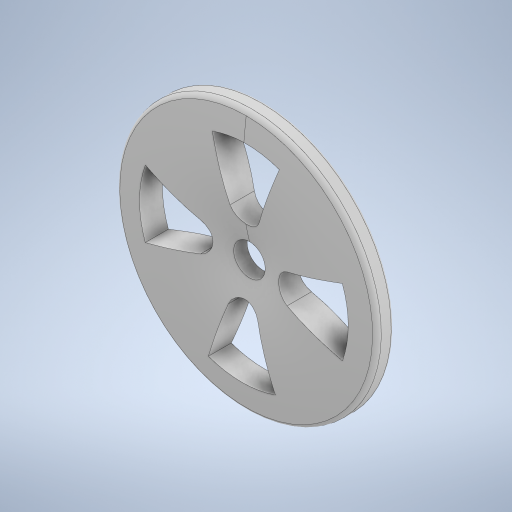
# Autodesk Inventor part: Anti tip wheels
Saved by Autodesk Inventor 2023 (Build 270158000, 158)
## iProperties
Created: 2023-11-13
Part Number: Anti tip wheels
Material: Generic
Document SubType Name: Modeling
Designer: Raghav
Density: 1 g/cm^3
Appearance: Default
Author: Raghav
Autodesk Inventor part; units mm, degrees
ref_plane "YZ Plane" through (0, 0, 0) normal (1, 0, 0) x (0, 1, 0)
ref_plane "XZ Plane" through (0, 0, 0) normal (0, 1, 0) x (-1, 0, 0)
ref_plane "XY Plane" through (0, 0, 0) normal (0, 0, 1) x (1, 0, 0)
sketch "Sketch1" plane through (0, 0, 0) normal (1, 0, 0) x (0, 1, 0)
  line L0 (52.3875, 0) -> (52.3875, 2)
  line L1 (52.3875, 0) -> (52.3875, -2)
  arc A0 (52.3875, 2) -> (50.9047, 4.0295) centre (50.2572, 2) ccw
  arc A1 (51.1141, -2.9824) -> (52.3875, -2) centre (51.3718, -2) ccw
  line L2 (50.9047, 4.0295) -> (25.8188, 7.012) construction
  line L3 (25.8188, 7.012) -> (16.2938, 5.4245) construction
  line L4 (16.2938, 5.4245) -> (-0.0182, 1.08) construction
  spline S0 degree 3 poles (50.9047, 4.0295) (25.8188, 7.012) (16.2938, 5.4245) (-0.0182, 1.08) knots 1 1 1 1 2 2 2 2
  line L5 (0, 0) -> (52.3875, 0)
  line L6 (51.1141, -2.9824) -> (25.8188, -7.012) construction
  line L7 (25.8188, -7.012) -> (16.2938, -5.4245) construction
  line L8 (16.2938, -5.4245) -> (-0.0182, -1.08) construction
  spline S1 degree 3 poles (51.1141, -2.9824) (25.8188, -7.012) (16.2938, -5.4245) (-0.0182, -1.08) knots 1 1 1 1 2 2 2 2
  line L9 (-0.0182, -1.08) -> (-0.0182, 1.08)
  dimension "d0" = 2
  dimension "d1" = 2
  constraints: 8 end point, 4 point on circle, 3 symmetric about line, 3 vertical, 2 centre point, 2 tangent, 1 horizontal, 6 other
  measures "d0" distance of L0.start L0.end
  measures "d1" distance of L0.start L1.end
revolve "Revolution1" add sketch "Sketch1" angle 360 about axis through (0, -0.0182, -1.08) along (0, 0, 1)
sketch "Sketch2" plane through (0, 0, 0) normal (0, 0, 1) x (1, 0, 0)
  circle A0 centre (0, 0) radius 6.35
  constraints: 1 centre point, 1 coincident
extrude "Extrusion1" cut sketch "Sketch2" along normal mid plane 105.25
sketch "Sketch3" plane through (0, 0, 0) normal (0, 0, 1) x (1, 0, 0)
  line L0 (0, 0) -> (-14.2875, -39.6875)
  arc A0 (-14.2875, -39.6875) -> (12.7, -39.6875) centre (-0.7937, -2.2049) ccw
  line L1 (12.7, -39.6875) -> (0, 0)
  line L2 (0, 0) -> (-6.2667, -17.4074)
  line L3 (5.588, -17.4625) -> (0, 0)
  arc A1 (5.588, -17.4625) -> (-6.2667, -17.4074) centre (-0.3491, -19.5378) ccw
  line L4 (39.6875, 12.7) -> (0, 0)
  arc A2 (39.6875, -14.2875) -> (39.6875, 12.7) centre (2.2049, -0.7937) ccw
  line L5 (0, 0) -> (39.6875, -14.2875)
  arc A3 (17.4625, 5.588) -> (17.4074, -6.2667) centre (19.5378, -0.3491) ccw
  line L6 (-12.7, 39.6875) -> (0, 0)
  arc A4 (14.2875, 39.6875) -> (-12.7, 39.6875) centre (0.7937, 2.2049) ccw
  line L7 (0, 0) -> (14.2875, 39.6875)
  arc A5 (-5.588, 17.4625) -> (6.2667, 17.4074) centre (0.3491, 19.5378) ccw
  line L8 (-39.6875, -12.7) -> (0, 0)
  arc A6 (-39.6875, 14.2875) -> (-39.6875, -12.7) centre (-2.2049, 0.7938) ccw
  line L9 (0, 0) -> (-39.6875, 14.2875)
  arc A7 (-17.4625, -5.588) -> (-17.4074, 6.2667) centre (-19.5378, 0.3491) ccw
  dimension "d13" = 360
  constraints: 20 end point, 16 point on circle, 12 point on line, 8 centre point, 2 coincident, 1 collinear, 1 tangent, 43 other
extrude "Extrusion3" cut sketch "Sketch3" along normal mid plane 105.25 contours A1 L1 A0 L0 | L4 A2 L5 A3 | L6 A4 L7 A5 | L8 A6 L9 A7
body "Solid1"
